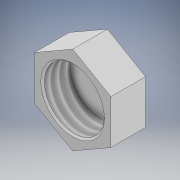
# Autodesk Inventor part: Wasserverteiler2
Saved by Autodesk Inventor 2021 (Build 250183000, 183)
## iProperties
Created: 2021-10-22
Part Number: Wasserverteiler2
Material: Generisch
Document SubType Name: Modeling
Designer: lukas
Density: 1 g/cm^3
Appearance: Vorgabe
Author: lukas
Autodesk Inventor part; units mm, degrees
ref_plane "YZ Plane" through (0, 0, 0) normal (1, 0, 0) x (0, 1, 0)
ref_plane "XZ Plane" through (0, 0, 0) normal (0, 1, 0) x (-1, 0, 0)
ref_plane "XY Plane" through (0, 0, 0) normal (0, 0, 1) x (1, 0, 0)
sketch "Skizze1" plane through (0, 0, 0) normal (0, 0, 1) x (1, 0, 0)
  line L0 (-15.4146, 0) -> (15.4146, 0) projected
  line L1 (0, -17.7824) -> (0, 17.7824) projected
  line L2 (-10.9895, 6.3689) -> (0.0209, 12.7017)
  line L3 (0.0209, 12.7017) -> (11.0104, 6.3328)
  line L4 (11.0104, 6.3328) -> (10.9895, -6.3689)
  line L5 (10.9895, -6.3689) -> (-0.0209, -12.7017)
  line L6 (-0.0209, -12.7017) -> (-11.0104, -6.3328)
  line L7 (-11.0104, -6.3328) -> (-10.9895, 6.3689)
  circle A0 centre (0, 0) radius 10
  dimension "d0" = 20
  dimension "d1" = 11
  constraints: 12 end point, 2 coincident, 1 centre point, 13 other
  measures "d0" diameter of A0
  measures "d1" distance from line of L4 A0.centre
extrude "Extrusion1" add sketch "Skizze1" along normal blind 10
sketch "Skizze2" plane through (0, 0, 10) normal (0, 0, 1) x (1, 0, 0)
  point P0 (0, 0)
hole "Bohrung1" at (0, 0, 10) direction (0, 0, -1) diameter 17.294 depth 8 thread size "M20x2.5" class "6H" standard "ISO Metric profile"
chamfer "Fase1" distance 0.5 angle 45 1 edges at (0, 8.647, 10)
